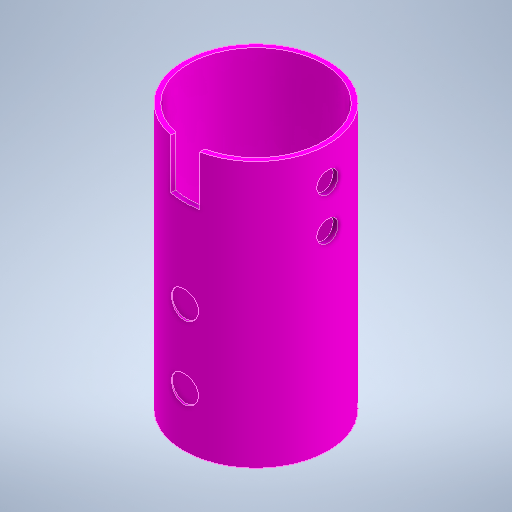
# Autodesk Inventor part: 1 part 27
Saved by Autodesk Inventor 2025.1 (Build 291241000, 241)
## iProperties
Created: 2024-08-01
Part Number: 1 part 27
Material: Generisch
Document SubType Name: Modeling
Designer: ffogue
Density: 1 g/cm^3
Appearance: Magenta
Author: ffogue
Autodesk Inventor part; units mm, degrees
sketch "Sketch1" plane through (0, 0, 0) normal (0, 0, 1) x (1, 0, 0)
  circle A0 centre (0, 0) radius 35
  circle A1 centre (0, 0) radius 37.5
  dimension "d1" = 70
  dimension "d36" = 75
  constraints: 2 centre point, 1 coincident
  measures "d1" diameter of A0
  measures "d36" diameter of A1
extrude "Extrusion1" add sketch "Sketch1" along normal blind 138
ref_plane "Work Plane2" through (0, -40, 0) normal (0, 1, 0) x (-1, 0, 0)
sketch "Sketch2" plane through (0, -40, 0) normal (0, 1, 0) x (-1, 0, 0)
  line L0 (37.5, 138) -> (-37.5, 138) projected
  line L1 (37.5, 0) -> (-37.5, 0) projected
  line L2 (7.5, 112) -> (-7.5, 112)
  line L3 (-7.5, 112) -> (-7.5, 138)
  line L4 (-7.5, 138) -> (7.5, 138)
  line L5 (7.5, 138) -> (7.5, 112)
  point P0 (0, 0)
  point P1 (0, 0)
  point P2 (0, 138)
  point P3 (-7.5, 125)
  point P4 (0, 112)
  dimension "d33" = 15
  dimension "d34" = 26
  constraints: 8 end point, 4 midpoint, 2 parallel, 1 horizontal, 1 perpendicular, 1 point on line, 1 vertical alignment
  measures "d33" distance from line of point (-7.5, 125) L5
  measures "d34" distance between parallel lines of L2 L0
extrude "Extrusion2" cut sketch "Sketch2" against normal up to surface round surface about axis through (0, 0, 0) along (0, 0, 1) radius 35 far side no
ref_plane "Work Plane3" through (37.5, 0, 0) normal (1, 0, 0) x (0, 1, 0)
sketch "Sketch3" plane through (37.5, 0, 0) normal (1, 0, 0) x (0, 1, 0)
  line L0 (-36.7423, 138) -> (-36.7423, 138) projected
  line L1 (37.5, 0) -> (-37.5, 0) projected
  line L2 (-37.5, 0) -> (-37.5, 112) projected
  line L3 (0, 138) -> (-37.5, 138) projected
  line L4 (-36.7423, 138) -> (-36.7423, 112) projected
  line L5 (-36.7423, 112) -> (-36.7423, 112) projected
  line L6 (-36.7423, 112) -> (-36.7423, 138) projected
  point P0 (0, 0)
  point P1 (39.2906, 138)
  point P2 (40, 0)
  point P3 (-40, 0)
  point P4 (0, 121)
  point P5 (0, 99)
  point P6 (0, 0)
  point P7 (-27.7633, 138)
  point P8 (40, 138)
  point P9 (-40, 138)
  dimension "d11" = 22
  dimension "d12" = 17
  constraints: 2 vertical alignment, 1 midpoint, 3 other
  measures "d11" distance of point (0, 121) point (0, 99)
  measures "d12" vertical distance of point (-27.763, 138) point (0, 121)
hole "Hole1" at (37.5, 0, 121) at (37.5, 0, 99) direction (-1, 0, 0) diameter 11 depth 3
ref_plane "Work Plane4" through (0, -40, 0) normal (0, -1, 0) x (1, 0, 0)
sketch "Sketch4" plane through (0, -40, 0) normal (0, -1, 0) x (1, 0, 0)
  line L0 (37.5, 138) -> (-37.5, 138) projected
  point P0 (0, 0)
  point P1 (0, 28)
  point P2 (0, 66)
  point P3 (40, 138)
  point P4 (40, 138)
  dimension "d21" = 38
  dimension "d35" = 28
  constraints: 2 vertical alignment
  measures "d21" distance of point (0, 66) point (0, 28)
  measures "d35" distance of point (0, 0) point (0, 28)
hole "Hole2" at (0, -40, 28) at (0, -40, 66) direction (0, 1, 0) diameter 14 depth 3.5
body "Solid1"
